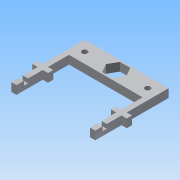
# Autodesk Inventor part: drieparts_assembly2
Saved by Autodesk Inventor 2015 (Build 190159000, 159)
## iProperties
Created: 2013-12-24
Part Number: drieparts_assembly2
Material: ABS Plastic
Document SubType Name: Modeling
Designer: aoki
Density: 1 g/cm^3
Appearance: Smooth - White
Author: aoki
Autodesk Inventor part; units mm, degrees
ref_plane "YZ Plane" through (0, 0, 0) normal (1, 0, 0) x (0, 1, 0)
ref_plane "XZ Plane" through (0, 0, 0) normal (0, 1, 0) x (-1, 0, 0)
ref_plane "XY Plane" through (0, 0, 0) normal (0, 0, 1) x (1, 0, 0)
sketch "Sketch1" plane through (0, 0, 0) normal (0, 0, 1) x (1, 0, 0)
  line L0 (40, -10) -> (-40, -10)
  line L1 (-40, -10) -> (-40, 10)
  line L2 (-40, 10) -> (40, 10)
  line L3 (40, 10) -> (40, -10)
  line L4 (0, -14) -> (0, 14) projected
  line L5 (40, -10) -> (30, -10)
  line L6 (-56, 0) -> (56, 0) projected
  circle A0 centre (-0.5449, 0.9437) radius 3.3235 projected
  line L7 (-4.875, -6.5563) -> (-9.2051, 0.9437) projected
  line L8 (-9.2051, 0.9437) -> (-4.875, 8.4437) projected
  line L9 (-4.875, 8.4437) -> (3.7853, 8.4437) projected
  line L10 (3.7853, 8.4437) -> (8.1154, 0.9437) projected
  line L11 (8.1154, 0.9437) -> (3.7853, -6.5563) projected
  line L12 (3.7853, -6.5563) -> (-4.875, -6.5563) projected
  circle A1 centre (-0.5449, 0.9437) radius 3.3235 projected
  line L13 (-4.875, -6.5563) -> (-9.2051, 0.9437) projected
  line L14 (-9.2051, 0.9437) -> (-4.875, 8.4437) projected
  line L15 (-4.875, 8.4437) -> (3.7853, 8.4437) projected
  line L16 (3.7853, 8.4437) -> (8.1154, 0.9437) projected
  line L17 (8.1154, 0.9437) -> (3.7853, -6.5563) projected
  line L18 (3.7853, -6.5563) -> (-4.875, -6.5563) projected
  point P0 (0, 0)
  dimension "d0" = 80
  dimension "d1" = 20
  dimension "d70" = 40
  dimension "d73" = 10
  constraints: 10 end point, 2 horizontal, 2 parallel, 1 perpendicular, 1 point on line
  measures "d0" distance of L1.end L2.end
  measures "d1" distance of L0.end L1.end
  measures "d70" distance between parallel lines of L3 L4
  measures "d73" distance between parallel lines of L2 L6
extrude "Extrusion1" add sketch "Sketch1" against normal blind 8
sketch "Sketch3" plane through (0, 0, 0) normal (0, 0, 1) x (1, 0, 0)
  line L0 (0, -14) -> (0, 14) projected
  line L1 (-56, 0) -> (56, 0) projected
  line L2 (-4.875, 8.4437) -> (4.875, 8.4437)
  line L3 (4.875, 8.4437) -> (9.75, 0)
  line L4 (9.75, 0) -> (4.875, -8.4437)
  line L5 (4.875, -8.4437) -> (-4.875, -8.4437)
  line L6 (-4.875, -8.4437) -> (-9.75, 0)
  line L7 (-9.75, 0) -> (-4.875, 8.4437)
  point P0 (0, 0)
  point P1 (0, 0)
  dimension "d65" = 19.5
  constraints: 12 end point, 1 coincident, 1 horizontal, 13 other
  measures "d65" distance of L3.end L6.end
extrude "Extrusion2" cut sketch "Sketch3" against normal blind 10
sketch "Sketch9" plane through (0, 0, -8) normal (0, 0, -1) x (-1, 0, 0)
  circle A0 centre (-30, 0) radius 2.6
  line L0 (0, -14) -> (0, 14) projected
  line L1 (56, 0) -> (-56, 0) projected
  circle A1 centre (30, 0) radius 2.6
  dimension "d40" = 5.2
  dimension "d41" = 60
  constraints: 2 centre point, 1 symmetric about line, 1 other
  measures "d40" diameter of A0
  measures "d41" distance of A1.centre A0.centre
extrude "Extrusion3" cut sketch "Sketch9" against normal through all
sketch "Sketch14" plane through (0, 0, 0) normal (0, 0, 1) x (1, 0, 0)
  circle A0 centre (30, 0) radius 2.6 projected
  circle A1 centre (-30, 0) radius 2.6 projected
  line L0 (-9.75, 0) -> (-4.875, 8.4437) projected
  line L1 (-4.875, 8.4437) -> (4.875, 8.4437) projected
  line L2 (4.875, 8.4437) -> (9.75, 0) projected
  line L3 (9.75, 0) -> (4.875, -8.4437) projected
  line L4 (4.875, -8.4437) -> (-4.875, -8.4437) projected
  line L5 (-4.875, -8.4437) -> (-9.75, 0) projected
  line L6 (40, -10) -> (-40, -10) projected
  line L7 (40, 10) -> (40, -10) projected
  line L8 (-40, 10) -> (40, 10) projected
  line L9 (-40, -10) -> (-40, 10) projected
  line L10 (-40, -10) -> (-35, -10)
  line L11 (-35, -10) -> (-35, -60)
  line L12 (-35, -60) -> (-40, -60)
  line L13 (-40, -60) -> (-40, -10)
  line L14 (-56, 0) -> (56, 0) projected
  line L15 (0, -33.313) -> (0, 17.2188) projected
  line L16 (40, -10) -> (35, -10)
  line L17 (35, -10) -> (35, -60)
  line L18 (35, -60) -> (40, -60)
  line L19 (40, -60) -> (40, -10)
  line L20 (-40, -30) -> (-45, -30)
  line L21 (-45, -30) -> (-45, -35)
  line L22 (-45, -35) -> (-40, -35)
  line L23 (-40, -35) -> (-40, -30)
  line L24 (-35, -30) -> (-30, -30)
  line L25 (-30, -30) -> (-30, -35)
  line L26 (-30, -35) -> (-35, -35)
  line L27 (-35, -35) -> (-35, -30)
  line L28 (40, -30) -> (45, -30)
  line L29 (45, -30) -> (45, -35)
  line L30 (45, -35) -> (40, -35)
  line L31 (40, -35) -> (40, -30)
  line L32 (35, -30) -> (30, -30)
  line L33 (30, -30) -> (30, -35)
  line L34 (30, -35) -> (35, -35)
  line L35 (35, -35) -> (35, -30)
  point P0 (0, 0)
  dimension "d74" = 5
  dimension "d75" = 50
  dimension "d78" = 5
  dimension "d79" = 5
  dimension "d80" = 5
  dimension "d81" = 20
  constraints: 48 end point, 11 symmetric about line, 6 parallel, 6 point on line, 3 horizontal, 3 perpendicular
  measures "d74" distance of L11.end L12.end
  measures "d75" distance of L12.end L6.end
  measures "d78" distance of L24.start L24.end
  measures "d79" distance of L20.start L20.end
  measures "d80" distance of L24.end L25.end
  measures "d81" distance between parallel lines of L6 L24
extrude "Extrusion8" add sketch "Sketch14" against normal blind 8 contours L19 L18 L17 L6 | L28 L29 L30 L19 | L17 L34 L33 L32 | L11 L12 L13 L6 | L24 L25 L26 L11 | L13 L22 L21 L20
sketch "Sketch15" plane through (-40, -60, 0) normal (-1, 0, 0) x (0, 0, 1)
  line L0 (0, 25) -> (-8, 25) projected
  line L1 (-8, 0) -> (-8, 25) projected
  line L2 (0, 0) -> (-8, 0) projected
  line L3 (0, 25) -> (0, 0) projected
  line L4 (0, 70) -> (0, 30) projected
  line L5 (0, 70) -> (-8, 70) projected
  line L6 (-8, 30) -> (-8, 70) projected
  line L7 (0, 30) -> (-8, 30) projected
  line L8 (0, 25) -> (-8, 25) projected
  line L9 (0, 30) -> (0, 25) projected
  line L10 (0, 30) -> (-8, 30) projected
  line L11 (-8, 25) -> (-8, 30) projected
  line L12 (0, 25) -> (-8, 25) projected
  line L13 (0, 11) -> (-4, 11)
  line L14 (-4, 11) -> (-4, 7)
  line L15 (-4, 7) -> (0, 7)
  line L16 (0, 7) -> (0, 11)
  point P0 (0, 60)
  dimension "d84" = 4
  dimension "d85" = 4
  dimension "d89" = 14
  constraints: 8 end point, 2 parallel, 1 horizontal, 1 perpendicular, 1 point on line
  measures "d84" distance of L14.end L15.end
  measures "d85" distance of L15.end L13.start
  measures "d89" distance between parallel lines of L0 L13
extrude "Extrusion9" cut sketch "Sketch15" against normal through all contours L3 L15 L14 L13
body "Solid1"
